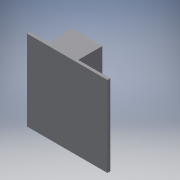
# Autodesk Inventor part: DCDriver
Saved by Autodesk Inventor 2017 (Build 210142000, 142)
## iProperties
Created: 2020-08-23
Part Number: DCDriver
Material: Generic
Document SubType Name: Modeling
Designer: agustin
Density: 1 g/cm^3
Appearance: Default
Author: agustin
Autodesk Inventor part; units mm, degrees
ref_plane "YZ Plane" through (0, 0, 0) normal (1, 0, 0) x (0, 1, 0)
ref_plane "XZ Plane" through (0, 0, 0) normal (0, 1, 0) x (-1, 0, 0)
ref_plane "XY Plane" through (0, 0, 0) normal (0, 0, 1) x (1, 0, 0)
sketch "Sketch1" plane through (0, 0, 0) normal (0, 1, 0) x (-1, 0, 0)
  line L0 (-43.2, 43.2) -> (43.2, 43.2)
  line L1 (43.2, 43.2) -> (43.2, -43.2)
  line L2 (43.2, -43.2) -> (-43.2, -43.2)
  line L3 (-43.2, -43.2) -> (-43.2, 43.2)
  line L4 (-43.2, 43.2) -> (43.2, -43.2) construction
  line L5 (43.2, 43.2) -> (-43.2, -43.2) construction
  point P0 (0, 0)
  dimension "d0" = 86.4
  dimension "d1" = 86.4
  constraints: 12 end point, 2 midpoint, 2 parallel, 1 horizontal, 1 perpendicular
  measures "d0" distance of L1.end L2.end
  measures "d1" distance of L0.end L1.end
extrude "Extrusion1" add sketch "Sketch1" along normal blind 3
sketch "Sketch2" plane through (0, 3, 0) normal (0, 1, 0) x (1, 0, 0)
  line L0 (-43.2, -43.2) -> (43.2, -43.2) projected
  line L1 (-43.2, -43.2) -> (-11.2, -43.2)
  line L2 (-11.2, -23) -> (-43.2, -23)
  line L3 (-43.2, -23) -> (-43.2, 23)
  line L4 (-43.2, 23) -> (-11.2, 23)
  line L5 (-11.2, 23) -> (-11.2, -23)
  line L6 (-11.2, -23) -> (-43.2, 23) construction
  line L7 (-43.2, -23) -> (-11.2, 23) construction
  point P0 (0, 0)
  point P1 (-27.2, 0)
  dimension "d5" = 46
  constraints: 14 end point, 2 horizontal, 2 midpoint, 2 parallel, 1 perpendicular
  measures "d5" distance of L2.end L3.end
extrude "Extrusion2" add sketch "Sketch2" along normal blind 46
scale "Scale1" factors (0.5, 0.5, 0.5) then translate (0, 0, 0) bodies 1
body "Solid1"
